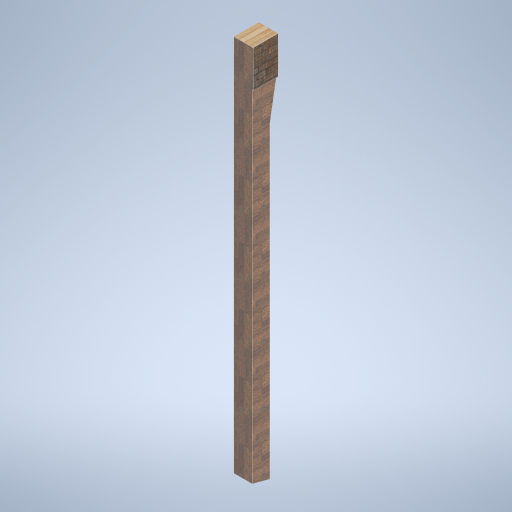
# Autodesk Inventor part: side_pillar_02
Saved by Autodesk Inventor 2024.2 (Build 282272000, 272)
## iProperties
Created: 2024-05-25
Part Number: side_pillar_02
Material: Wood (Maple)
Document SubType Name: Modeling
Designer: LOSTER_1
Density: 0.67 g/cm^3
Appearance: Natural Maple - Glossy Dark Tint
Author: LOSTER_1
Autodesk Inventor part; units mm, degrees
ref_plane "YZ Plane" through (0, 0, 0) normal (1, 0, 0) x (0, 1, 0)
ref_plane "XZ Plane" through (0, 0, 0) normal (0, 1, 0) x (-1, 0, 0)
ref_plane "XY Plane" through (0, 0, 0) normal (0, 0, 1) x (1, 0, 0)
sketch "Sketch2" plane through (0, 0, 0) normal (1, 0, 0) x (0, 1, 0)
  line L0 (17266.7168, -4180.2603) -> (17266.7177, -4180.2555)
  line L1 (21684.5168, -7422.7726) -> (21684.5142, -2804.0577)
  arc A0 (17539.1028, -4226.3631) -> (17589.5175, -4034.0683) centre (-21127.9015, 6013.8899) ccw
  line L2 (17539.1028, -4226.3631) -> (17839.1028, -4226.363)
  line L3 (17839.1028, -4226.363) -> (17839.1027, -4034.0682)
  line L4 (17839.1027, -4034.0682) -> (17589.5175, -4034.0683)
  line L5 (17839.1027, -4034.0682) -> (21684.5149, -4034.0659)
  line L6 (17839.1028, -4226.363) -> (21684.515, -4226.3608)
  line L7 (20884.515, -4226.3612) -> (21278.4381, -4295.8205)
  line L8 (20884.515, -4226.3612) -> (21284.515, -4226.3612) construction
  line L9 (21278.4381, -4295.8205) -> (21278.4381, -3784.3997)
  line L10 (20884.515, -4034.0664) -> (21278.4381, -3964.6071)
  line L11 (20884.515, -4034.0664) -> (21284.515, -4034.0664) construction
  line L12 (21278.4381, -3964.6071) -> (21278.4381, -3954.6071)
  line L13 (21278.4381, -3954.6071) -> (21684.5148, -3954.6069)
  line L14 (21278.4381, -4295.8205) -> (21278.4381, -4305.8205)
  line L15 (21278.4381, -4305.8205) -> (21684.515, -4305.8203)
  point P0 (0, 0)
  dimension "d0" = 40000
  dimension "d1" = 300
  dimension "d5" = 400
  dimension "d6" = 10
  dimension "d7" = 10
  dimension "d8" = 10
  dimension "d9" = 10
  constraints: 32 end point, 7 perpendicular, 7 point on line, 2 equal length, 2 horizontal, 2 point on circle, 2 vertical, 1 centre point
  measures "d0" radius of A0
  measures "d1" distance of L2.start L2.end
  measures "d5" distance of L7.start L7.end
  measures "d6" angle of L7 L8
  measures "d7" angle of L11 L10
  measures "d8" distance of L10.end L12.end
  measures "d9" distance of L7.end L14.end
extrude "Extrusion1" add sketch "Sketch2" along normal blind 200 contours L15 L14 L9 L6 L1 | L6 L9 L5 L1 | L9 L7 L6 | L6 L3 L5 L9 | L2 A0 L4 L3
sketch "Sketch3" plane through (200, 0, 0) normal (1, 0, 0) x (0, 0, -1)
  line L0 (4305.8203, 21684.515) -> (4034.0659, 21684.5149) projected
  line L1 (4305.8205, 21278.4381) -> (4034.0659, 21278.4381)
  line L2 (4034.0659, 21278.4381) -> (4034.0659, 21684.5149)
  line L3 (4034.0659, 21684.5149) -> (4305.8205, 21684.5149)
  line L4 (4305.8205, 21684.5149) -> (4305.8205, 21278.4381)
  point P0 (0, 0)
  constraints: 8 end point, 2 parallel, 1 horizontal, 1 perpendicular
extrude "Extrusion2" add sketch "Sketch3" along normal blind 10
body "Solid1"
